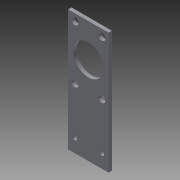
# Autodesk Inventor part: upper pulley mount
Saved by Autodesk Inventor 2013 (Build 170138000, 138)
## iProperties
Created: 2013-01-20
Part Number: upper pulley mount
Material: Generic
Document SubType Name: Sheet Metal
Designer: Arpan
Density: 1 g/cm^3
Sheet Metal Rule: Default
Author: Arpan
Autodesk Inventor part; units mm, degrees
ref_plane "YZ Plane" through (0, 0, 0) normal (1, 0, 0) x (0, 1, 0)
ref_plane "XZ Plane" through (0, 0, 0) normal (0, 1, 0) x (-1, 0, 0)
ref_plane "XY Plane" through (0, 0, 0) normal (0, 0, 1) x (1, 0, 0)
sketch "Sketch1" plane through (0, 0, 0) normal (0, 0, 1) x (1, 0, 0)
  line L0 (0, 0) -> (-38.1, 0)
  line L1 (0, 0) -> (0, 114.3)
  line L2 (0, 114.3) -> (-38.1, 114.3)
  line L3 (-38.1, 114.3) -> (-38.1, 0)
  line L4 (-38.1, 114.3) -> (-31.75, 114.3)
  line L5 (-31.75, 114.3) -> (-31.75, 12.7)
  line L6 (0, 114.3) -> (-6.35, 114.3)
  line L7 (-6.35, 114.3) -> (-6.35, 12.7)
  circle A0 centre (-31.75, 12.7) radius 2.1463
  circle A1 centre (-6.35, 12.7) radius 2.1463
  dimension "d0" = 38.1
  dimension "d1" = 114.3
  dimension "d2" = 6.35
  dimension "d3" = 101.6
  dimension "d4" = 6.35
  dimension "d5" = 4.2926
  dimension "d6" = 4.2926
  dimension "d7" = 101.6
  measures "d0" distance of L0.start L0.end
  measures "d1" distance of L0.start L1.end
  measures "d2" distance of L2.end L4.end
  measures "d3" distance of L4.end L5.end
  measures "d4" distance of L1.end L6.end
  measures "d5" diameter of A0
  measures "d6" diameter of A1
  measures "d7" distance of L6.end L7.end
extrude "Plate1" add sketch "Sketch1" along normal blind 3.175
sketch "Sketch3" plane through (0, 0, 3.175) normal (0, 0, 1) x (1, 0, 0)
  line L0 (0, 114.3) -> (0, 0) projected
  line L1 (-38.1, 114.3) -> (0, 114.3) projected
  line L2 (-38.1, 0) -> (-38.1, 114.3) projected
  line L3 (-38.1, 114.3) -> (-38.1, 107.95)
  line L4 (-38.1, 107.95) -> (-31.75, 107.95)
  circle A0 centre (-31.75, 107.95) radius 3.3782
  line L5 (0, 114.3) -> (0, 107.95)
  line L6 (0, 107.95) -> (-6.35, 107.95)
  circle A1 centre (-6.35, 107.95) radius 3.3782
  line L7 (-38.1, 107.95) -> (-38.1, 57.15)
  line L8 (-38.1, 57.15) -> (-31.75, 57.15)
  line L9 (0, 57.15) -> (-6.35, 57.15)
  circle A2 centre (-31.75, 57.15) radius 3.3782
  circle A3 centre (-6.35, 57.15) radius 3.3782
  line L10 (-38.1, 114.3) -> (-38.1, 82.55)
  line L11 (-38.1, 82.55) -> (-19.05, 82.55)
  circle A4 centre (-19.05, 82.55) radius 14.2875
  dimension "d19" = 6.35
  dimension "d20" = 6.35
  dimension "d21" = 6.7564
  dimension "d22" = 6.35
  dimension "d23" = 6.35
  dimension "d24" = 6.7564
  dimension "d25" = 50.8
  dimension "d26" = 6.35
  dimension "d27" = 6.35
  dimension "d28" = 57.15
  dimension "d29" = 6.7564
  dimension "d30" = 6.7564
  dimension "d31" = 31.75
  dimension "d32" = 28.575
  constraints: 18 end point, 5 centre point, 5 coincident, 4 perpendicular, 3 midpoint, 2 point on line, 1 collinear
  measures "d19" distance of L1.start L3.end
  measures "d20" distance of L3.end L4.end
  measures "d21" diameter of A0
  measures "d22" distance of L0.start L5.end
  measures "d23" distance of L5.end L6.end
  measures "d24" diameter of A1
  measures "d25" distance of L3.end L7.end
  measures "d26" distance of L7.end L8.end
  measures "d27" distance of L9.start L9.end
  measures "d28" distance between parallel lines of L1 L9
  measures "d29" diameter of A2
  measures "d30" diameter of A3
  measures "d31" distance of L1.start L10.end
  measures "d32" diameter of A4
extrude "Cut1" cut sketch "Sketch3" against normal blind 3.175
equation "\"d33\" = Thickness"
equation "\"BendRadius\" = Thickness"
equation "\"BendReliefWidth\" = Thickness"
equation "\"BendReliefDepth\" = 0.5 * Thickness"
equation "\"CornerReliefSize\" = 4 * Thickness"
equation "\"MinimumRemnant\" = 2 * Thickness"
equation "\"TransitionRadius\" = BendRadius"
equation "\"JacobiRadiusSize\" = BendRadius"
equation "\"GapSize\" = Thickness"
equation "\"d8\" = BendRadius"
equation "\"Thickness\" = 3.175"
body "Solid1"
